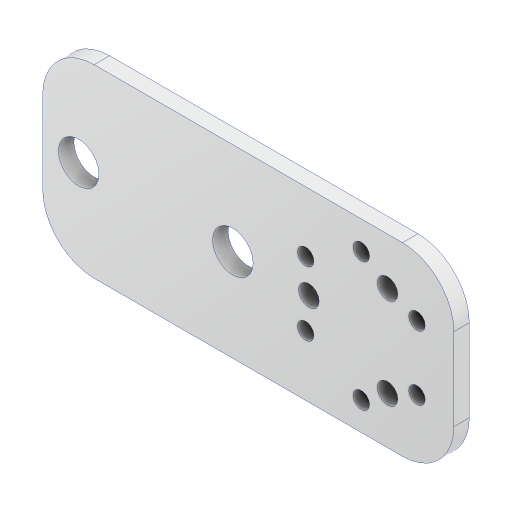
# Autodesk Inventor part: link_plate
Saved by Autodesk Inventor 2024.3 (Build 283343000, 343)
## iProperties
Created: 2024-10-12
Part Number: link_plate
Material: アルミニウム 6061
Document SubType Name: Sheet Metal
Designer: haya
Density: 2.7 g/cm^3
Sheet Metal Rule: Default_mm
Appearance: アルミニウム - フラット
Mass: 24.1844 g
Surface Area: 70.3203 cm^2
Volume: 8.95719 cm^3
Author: haya
Autodesk Inventor part; units mm, degrees
ref_plane "YZ Plane" through (0, 0, 0) normal (1, 0, 0) x (0, 1, 0)
ref_plane "XZ Plane" through (0, 0, 0) normal (0, 1, 0) x (-1, 0, 0)
ref_plane "XY Plane" through (0, 0, 0) normal (0, 0, 1) x (1, 0, 0)
sketch "スケッチ1" plane through (0, 0, 0) normal (0, 0, 1) x (1, 0, 0)
  line L0 (-40, 18) -> (40, 18)
  line L1 (40, 18) -> (40, -18)
  line L2 (40, -18) -> (-40, -18)
  line L3 (-40, -18) -> (-40, 18)
  line L4 (0, 0) -> (0, 18) construction
  line L5 (0, 0) -> (40, 0) construction
  dimension "d0" = 36
  dimension "d1" = 80
  measures "d0" distance of L0.end L1.end
  measures "d1" distance of L0.start L0.end
extrude "プレート1" add sketch "スケッチ1" along normal blind 3
sketch "スケッチ2" plane through (0, 0, 3) normal (0, 0, 1) x (1, 0, 0)
  line L0 (40, 18) -> (40, -18) projected
  line L1 (-40, 18) -> (-40, -18) projected
  line L2 (-40, 0) -> (40, 0) construction
  point P0 (22, 0)
  point P1 (11.8, 0)
  point P2 (27.1, -8.8335)
  point P3 (27.1, 8.8335)
  dimension "d3" = 10.2
  dimension "d6" = 360
  dimension "d116" = 18
  constraints: 2 end point, 2 midpoint, 1 point on line, 4 other
  measures "d3" distance of point (11.8, 0) point (22, 0)
  measures "d116" distance from line of point (22, 0) L0
hole "穴1" at (11.8, 0, 3) at (27.1, -8.8335, 3) at (27.1, 8.8335, 3) direction (0, 0, -1) diameter 4 depth 3 tip angle 118
sketch "スケッチ3" plane through (0, 0, 3) normal (0, 0, 1) x (1, 0, 0)
  line L0 (40, 18) -> (40, -18) projected
  point P0 (22, 0)
  point P1 (22, -12.5)
  point P2 (32.8253, -6.25)
  point P3 (32.8253, 6.25)
  point P4 (22, 12.5)
  point P5 (11.1747, 6.25)
  point P6 (11.1747, -6.25)
  dimension "d15" = 12.5
  dimension "d18" = 360
  dimension "d117" = 18
  constraints: 7 other
  measures "d15" distance of point (22, -12.5) point (22, 0)
  measures "d117" distance from line of point (22, 0) L0
hole "穴2" at (22, -12.5, 3) at (32.8253, -6.25, 3) at (32.8253, 6.25, 3) at (22, 12.5, 3) at (11.1747, 6.25, 3) at (11.1747, -6.25, 3) direction (0, 0, -1) diameter 3.2 depth 3 tip angle 118
sketch "スケッチ13" plane through (0, 0, 0) normal (0, 0, -1) x (-1, 0, 0)
  line L0 (0, 0) -> (40, 0) construction
  line L1 (40, -18) -> (40, 18) projected
  line L2 (-40, 18) -> (-40, -18) projected
  point P0 (33, 0)
  point P1 (3, 0)
  dimension "d127" = 30
  dimension "d128" = 43
  constraints: 2 end point, 2 point on line, 1 midpoint
  measures "d127" distance of point (33, 0) point (3, 0)
  measures "d128" distance from line of point (3, 0) L2
hole "穴10" at (-33, 0, 0) at (-3, 0, 0) direction (0, 0, 1) diameter 7.9 depth 3 tip angle 118
fillet "フィレット1" radius 10 4 edges at (40, -18, 1.5) (40, 18, 1.5) (-40, 18, 1.5) (-40, -18, 1.5)
equation "\"d13\" = d3"
equation "\"d125\" = Thickness"
equation "\"d2\" = Thickness"
equation "\"BendRadius\" = Thickness"
equation "\"BendReliefWidth\" = Thickness"
equation "\"BendReliefDepth\" = 0.5 * Thickness"
equation "\"CornerReliefSize\" = 4 * Thickness"
equation "\"MinimumRemnant\" = 2 * Thickness"
equation "\"TransitionRadius\" = BendRadius"
equation "\"JacobiRadiusSize\" = BendRadius"
equation "\"GapSize\" = Thickness"
equation "\"Thickness\" = 3"
